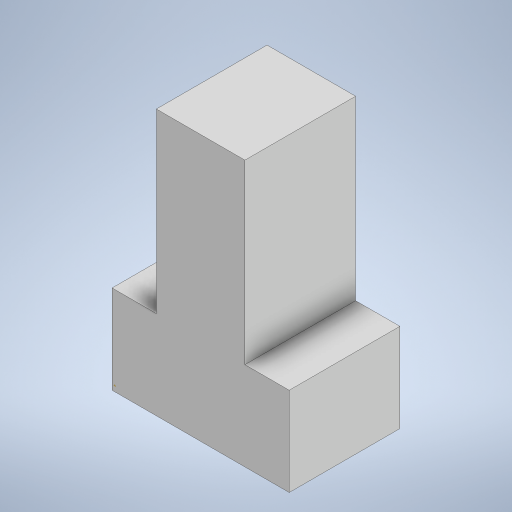
# Autodesk Inventor part: BT003_Prisma
Saved by Autodesk Inventor 2023 (Build 270158000, 158)
## iProperties
Created: 2022-04-26
Part Number: BT003_Prisma
Material: Generic
Document SubType Name: Modeling
Designer: Altar
Density: 1 g/cm^3
Appearance: Default
Author: Altar
Autodesk Inventor part; units mm, degrees
ref_plane "YZ Plane" through (0, 0, 0) normal (1, 0, 0) x (0, 1, 0)
ref_plane "XZ Plane" through (0, 0, 0) normal (0, 1, 0) x (-1, 0, 0)
ref_plane "XY Plane" through (0, 0, 0) normal (0, 0, 1) x (1, 0, 0)
sketch "Sketch1" plane through (0, 0, 0) normal (0, 0, 1) x (1, 0, 0)
  line L0 (-0.625, -1.25) -> (-0.625, 18.75)
  line L1 (-0.625, 18.75) -> (9.375, 18.75)
  line L2 (9.375, 18.75) -> (9.375, 58.75)
  line L3 (9.375, 58.75) -> (29.375, 58.75)
  line L4 (29.375, 58.75) -> (29.375, 18.75)
  line L5 (29.375, 18.75) -> (39.375, 18.75)
  line L6 (39.375, 18.75) -> (39.375, -1.25)
  line L7 (39.375, -1.25) -> (-0.625, -1.25)
  point P0 (0, 0)
  dimension "d0" = 40
  dimension "d1" = 40
  dimension "d2" = 20
  dimension "d3" = 10
  dimension "d4" = 10
  dimension "d5" = 20
  constraints: 16 end point, 6 perpendicular, 1 horizontal, 1 point on line, 1 vertical
  measures "d0" distance of L1.end L2.end
  measures "d1" distance of L6.end L0.start
  measures "d2" distance of L2.end L3.end
  measures "d3" distance of L4.end L5.end
  measures "d4" distance of L0.end L1.end
  measures "d5" distance of L0.start L0.end
extrude "Extrusion1" add sketch "Sketch1" against normal blind 25
body "Solid1"
